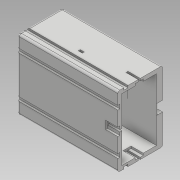
# Autodesk Inventor part: case
Saved by Autodesk Inventor 2018.2 (Build 222227000, 227)
## iProperties
Created: 2019-05-28
Part Number: case
Material: Generico
Document SubType Name: Modeling
Designer: fabio
Density: 1 g/cm^3
Appearance: Default
Author: fabio
Autodesk Inventor part; units mm, degrees
ref_plane "YZ Plane" through (0, 0, 0) normal (1, 0, 0) x (0, 1, 0)
ref_plane "XZ Plane" through (0, 0, 0) normal (0, 1, 0) x (-1, 0, 0)
ref_plane "XY Plane" through (0, 0, 0) normal (0, 0, 1) x (1, 0, 0)
sketch "Schizzo1" plane through (0, 0, 0) normal (0, 1, 0) x (-1, 0, 0)
  line L0 (-20.2, 15.3) -> (20.2, 15.3)
  line L1 (20.2, 15.3) -> (20.2, -15.3)
  line L2 (20.2, -15.3) -> (-20.2, -15.3)
  line L3 (-20.2, -15.3) -> (-20.2, 15.3)
  line L4 (-20.2, 15.3) -> (20.2, -15.3) construction
  line L5 (20.2, 15.3) -> (-20.2, -15.3) construction
  line L6 (20.2, 13.3) -> (-20.2, 13.3)
  line L7 (20.2, 2.3) -> (20.2, 15.3)
  line L8 (20.2, 15.3) -> (15.7, 15.3)
  line L9 (15.7, 15.3) -> (15.7, 2.3)
  line L10 (15.7, 2.3) -> (20.2, 2.3)
  line L11 (20.2, -9.3) -> (20.2, -15.3)
  line L12 (20.2, -15.3) -> (15.7, -15.3)
  line L13 (15.7, -15.3) -> (15.7, -9.3)
  line L14 (15.7, -9.3) -> (20.2, -9.3)
  line L15 (20.2, 15.3) -> (20.2, 12.3)
  line L16 (20.2, 12.3) -> (2.7, 12.3)
  line L17 (2.7, 12.3) -> (2.7, 15.3)
  line L18 (2.7, 15.3) -> (20.2, 15.3)
  point P0 (0, 0)
  dimension "d0" = 40.4
  dimension "d1" = 30.6
  dimension "d2" = 2
  dimension "d3" = 4.5
  dimension "d4" = 13
  dimension "d5" = 4.5
  dimension "d6" = 6
  dimension "d19" = 3
  dimension "d20" = 17.5
  constraints: 38 end point, 8 parallel, 7 perpendicular, 5 point on line, 2 midpoint, 1 horizontal
  measures "d0" distance of L1.end L2.end
  measures "d1" distance of L2.end L0.start
  measures "d2" distance between parallel lines of L6 L0
  measures "d3" distance of L9.end L7.start
  measures "d4" distance of L8.end L9.end
  measures "d5" distance of L13.end L11.start
  measures "d6" distance of L12.end L13.end
  measures "d19" distance of L16.end L17.end
  measures "d20" distance between parallel lines of L17 L7
extrude "Estrusione1" add sketch "Schizzo1" along normal mid plane 4 contours L0 L17 L6 L3 | L0 L9 L6 L17 | L0 L1 L6 L9 | L6 L9 L16 L17 | L6 L1 L16 L9 | L13 L14 L1 L2 | L16 L1 L10 L9
sketch "Schizzo6" plane through (-20.2, 2, 15.3) normal (0, 0, 1) x (1, 0, 0)
  line L0 (0, 0) -> (0, -4) projected
  line L1 (40.4, 0) -> (40.4, -4) projected
  line L2 (0, -4) -> (0, 0) projected
  line L3 (40.4, -3) -> (0, -3)
  line L4 (0, -3) -> (0, -1)
  line L5 (0, -1) -> (40.4, -1)
  line L6 (40.4, -1) -> (40.4, -3)
  line L7 (40.4, -3) -> (0, -1) construction
  line L8 (0, -3) -> (40.4, -1) construction
  point P0 (20.2, -2)
  dimension "d111" = 2
  constraints: 12 end point, 2 midpoint, 2 parallel, 1 horizontal, 1 perpendicular, 1 point on line
  measures "d111" distance between parallel lines of L3 L5
extrude "Estrusione5" cut sketch "Schizzo6" against normal up to surface (30.6 mm away)
sketch "Schizzo7" plane through (0, 2, 0) normal (0, 1, 0) x (1, 0, 0)
  line L0 (-20.2, -15.3) -> (20.2, -15.3) projected
  line L1 (-20.2, -2.3) -> (-20.2, -15.3) projected
  line L2 (-20.2, 15.3) -> (-20.2, 9.3) projected
  line L3 (-15.7, 15.3) -> (-20.2, 15.3) projected
  line L4 (20.2, -15.3) -> (-20.2, -15.3) projected
  line L5 (-20.2, -15.3) -> (20.2, -15.3)
  line L6 (20.2, -15.3) -> (20.2, -17.3)
  line L7 (20.2, -17.3) -> (-20.2, -17.3)
  line L8 (-20.2, -17.3) -> (-20.2, -15.3)
  line L9 (20.2, -13.3) -> (-2.7, -13.3) projected
  line L10 (-20.2, 15.3) -> (-15.7, 15.3) projected
  line L11 (-20.2, 15.3) -> (20.2, 15.3)
  line L12 (20.2, 15.3) -> (20.2, 17.3)
  line L13 (20.2, 17.3) -> (-20.2, 17.3)
  line L14 (-20.2, 17.3) -> (-20.2, 15.3)
  line L15 (-20.2, -17.3) -> (-20.2, 17.3)
  line L16 (-20.2, 17.3) -> (-22.2, 17.3)
  line L17 (-22.2, 17.3) -> (-22.2, -17.3)
  line L18 (-22.2, -17.3) -> (-20.2, -17.3)
  point P0 (0, 0)
  dimension "d25" = 2
  dimension "d26" = 2
  dimension "d27" = 2
  constraints: 24 end point, 7 parallel, 3 perpendicular, 2 collinear
  measures "d25" distance of L0.end L6.end
  measures "d26" distance of L11.end L12.end
  measures "d27" distance of L13.end L16.end
extrude "Estrusione6" add sketch "Schizzo7" against normal up to surface (4 mm away)
sketch "Schizzo10" plane through (-20.2, 2, 2.3) normal (1, 0, 0) x (0, 0, -1)
  line L0 (11.6, -4) -> (11.6, -3) projected
  line L1 (11.6, -4) -> (11.6, -3)
  line L2 (11.6, -3) -> (9.6, -3)
  line L3 (9.6, -3) -> (9.6, -4)
  line L4 (9.6, -4) -> (11.6, -4)
  line L5 (11.6, -3) -> (17.6, -3) projected
  point P0 (2.3, -2)
  dimension "d33" = 2
  dimension "d130" = 1
  constraints: 8 end point, 2 parallel, 2 point on line, 1 perpendicular, 2 other
  measures "d33" distance of L3.end L1.start
  measures "d130" distance of L2.end L3.end
extrude "Estrusione8" cut sketch "Schizzo10" against normal up to surface (2 mm away)
sketch "Schizzo12" plane through (-22.2, 2, 17.3) normal (0, 0, 1) x (1, 0, 0)
  line L0 (42.4, 0) -> (42.4, -4) projected
  line L1 (42.4, 0) -> (42.4, -4) projected
  line L2 (22.4, -3) -> (24.4, -3)
  line L3 (24.4, -3) -> (24.4, -4)
  line L4 (24.4, -4) -> (22.4, -4)
  line L5 (22.4, -4) -> (22.4, -3)
  line L6 (42.4, -3) -> (2, -3) projected
  point P0 (22.2, -2)
  dimension "d42" = 18
  dimension "d43" = 2
  dimension "d44" = 1
  constraints: 8 end point, 2 parallel, 1 horizontal, 1 perpendicular, 1 other
  measures "d42" distance between parallel lines of L0 L3
  measures "d43" distance of L3.end L4.end
  measures "d44" distance of L4.end L2.start
extrude "Estrusione10" cut sketch "Schizzo12" against normal up to surface (4 mm away)
sketch "Schizzo13" plane through (20.2, 1, 13.3) normal (1, 0, 0) x (0, 0, -1)
  line L0 (-4, 1) -> (0, 1) projected
  line L1 (28.6, 1) -> (30.6, 1) projected
  line L2 (-4, 1) -> (-4, -3) projected
  line L3 (-2, 0) -> (-2, -2) projected
  line L4 (-4, 1) -> (-2, 1)
  line L5 (-2, 1) -> (-2, 8.5)
  line L6 (-2, 8.5) -> (-4, 8.5)
  line L7 (-4, 8.5) -> (-4, 1)
  line L8 (-2, -2) -> (-2, 1)
  line L9 (22.6, 1) -> (28.6, 1) projected
  line L10 (28.6, 1) -> (30.6, 1)
  line L11 (30.6, 1) -> (30.6, 8.5)
  line L12 (30.6, 8.5) -> (28.6, 8.5)
  line L13 (28.6, 8.5) -> (28.6, 1)
  line L14 (-4, 8.5) -> (30.6, 8.5)
  line L15 (30.6, 8.5) -> (30.6, 11.5)
  line L16 (30.6, 11.5) -> (-4, 11.5)
  line L17 (-4, 11.5) -> (-4, 8.5)
  point P0 (13.3, -1)
  dimension "d47" = 10.5
  dimension "d48" = 3
  constraints: 26 end point, 6 parallel, 4 perpendicular, 2 collinear, 1 midpoint
  measures "d47" distance from line of L3.end L6
  measures "d48" distance of L11.end L15.end
extrude "Estrusione11" add sketch "Schizzo13" against normal up to surface (42.4 mm away)
sketch "Schizzo15" plane through (20.2, -2, 13.3) normal (1, 0, 0) x (0, 0, -1)
  line L0 (0, 0) -> (-4, 0) projected
  line L1 (-2, 3) -> (-2, 1) projected
  line L2 (28.6, 0) -> (30.6, 0) projected
  line L3 (-4, 0) -> (-2, 0)
  line L4 (-2, 0) -> (-2, -5.5)
  line L5 (-2, -5.5) -> (-4, -5.5)
  line L6 (-4, -5.5) -> (-4, 0)
  line L7 (-2, 1) -> (-2, 0)
  line L8 (28.6, 11.5) -> (28.6, 0) projected
  line L9 (28.6, 0) -> (30.6, 0)
  line L10 (30.6, 0) -> (30.6, -5.5)
  line L11 (30.6, -5.5) -> (28.6, -5.5)
  line L12 (28.6, -5.5) -> (28.6, 0)
  line L13 (-4, -5.5) -> (30.6, -5.5)
  line L14 (30.6, -5.5) -> (30.6, -7.5)
  line L15 (30.6, -7.5) -> (-4, -7.5)
  line L16 (-4, -7.5) -> (-4, -5.5)
  point P0 (13.3, 2)
  dimension "d53" = 8.5
  dimension "d54" = 2
  constraints: 26 end point, 6 parallel, 4 perpendicular, 2 collinear, 1 midpoint
  measures "d53" distance from line of L5 L1.start
  measures "d54" distance of L10.end L14.end
extrude "Estrusione13" add sketch "Schizzo15" against normal up to surface (42.4 mm away)
sketch "Schizzo14" plane through (0, 2, 0) normal (0, 1, 0) x (1, 0, 0)
  line L0 (-22.2, 15.3) -> (-22.2, -15.3) projected
  line L1 (-15.7, 15.3) -> (-22.2, 15.3) projected
  line L2 (-22.2, -15.3) -> (20.2, -15.3) projected
  line L3 (-20.2, -2.3) -> (-20.2, 9.3) projected
  line L4 (-22.2, 15.3) -> (-22.2, -15.3)
  line L5 (-22.2, -15.3) -> (-20.2, -15.3)
  line L6 (-20.2, -15.3) -> (-20.2, 15.3)
  line L7 (-20.2, 15.3) -> (-22.2, 15.3)
  point P0 (0, 0)
  constraints: 8 end point, 3 equal length, 1 collinear, 1 perpendicular
extrude "Estrusione14" add sketch "Schizzo14" along normal up to surface (7.5 mm away)
sketch "Schizzo16" plane through (0, -2, 0) normal (0, -1, 0) x (1, 0, 0)
  line L0 (-22.2, -15.3) -> (-22.2, 15.3) projected
  line L1 (-20.2, 2.3) -> (-20.2, -7.3) projected
  line L2 (-22.2, -15.3) -> (-15.7, -15.3) projected
  line L3 (20.2, 15.3) -> (-22.2, 15.3) projected
  line L4 (-22.2, -15.3) -> (-22.2, 15.3)
  line L5 (-22.2, 15.3) -> (-20.2, 15.3)
  line L6 (-20.2, 15.3) -> (-20.2, -15.3)
  line L7 (-20.2, -15.3) -> (-22.2, -15.3)
  point P0 (0, 0)
  point P1 (-20.2, -9.2)
  constraints: 8 end point, 2 parallel, 1 collinear, 1 perpendicular, 1 vertical
extrude "Estrusione15" add sketch "Schizzo16" along normal up to surface (5.5 mm away)
sketch "Schizzo20" plane through (20.2, 12.5, 17.3) normal (1, 0, 0) x (0, 0, -1)
  line L0 (34.6, 0) -> (0, 0) projected
  line L1 (0, 0) -> (0, -22) projected
  line L2 (0, -22) -> (34.6, -22) projected
  line L3 (32.6, -20) -> (2, -20) projected
  line L4 (2, -20) -> (2, -14.5) projected
  line L5 (2, -10.5) -> (2, -3) projected
  line L6 (2, -3) -> (32.6, -3) projected
  line L7 (32.6, -3) -> (32.6, -20) projected
  line L8 (34.6, -22) -> (34.6, 0) projected
  line L9 (2, -10.5) -> (2, -14.5)
  point P0 (17.3, -12.5)
  constraints: 2 end point
extrude "Estrusione17" add sketch "Schizzo20" along normal blind 7
sketch "Schizzo26" plane through (27.2, 12.5, 17.3) normal (1, 0, 0) x (0, 0, -1)
  line L0 (2, -3) -> (32.6, -3) projected
  line L1 (2, -20) -> (2, -3) projected
  line L2 (32.6, -20) -> (2, -20) projected
  line L3 (32.6, -3) -> (32.6, -20) projected
  line L4 (2, -3) -> (32.6, -3) projected
  line L5 (17.3, -3) -> (17.3, -20)
  line L6 (32.6, -20) -> (2, -20) projected
  line L7 (2, -11.5) -> (17.3, -11.5)
  line L8 (17.3, -11.5) -> (32.6, -11.5)
  line L9 (17.8, -3) -> (16.8, -3)
  line L10 (16.8, -3) -> (16.8, -2)
  line L11 (16.8, -2) -> (15.3, -2)
  line L12 (15.3, -2) -> (15.3, -1)
  line L13 (15.3, -1) -> (19.3, -1)
  line L14 (19.3, -1) -> (19.3, -2)
  line L15 (19.3, -2) -> (17.8, -2)
  line L16 (17.8, -2) -> (17.8, -3)
  line L17 (17.8, -20) -> (16.8, -20)
  line L18 (16.8, -20) -> (16.8, -21)
  line L19 (16.8, -21) -> (15.3, -21)
  line L20 (15.3, -21) -> (15.3, -22)
  line L21 (15.3, -22) -> (19.3, -22)
  line L22 (19.3, -22) -> (19.3, -21)
  line L23 (19.3, -21) -> (17.8, -21)
  line L24 (17.8, -21) -> (17.8, -20)
  line L25 (32.6, -13.5) -> (32.6, -9.5)
  line L26 (32.6, -9.5) -> (33.6, -9.5)
  line L27 (33.6, -9.5) -> (33.6, -11)
  line L28 (33.6, -11) -> (34.6, -11)
  line L29 (34.6, -11) -> (34.6, -12)
  line L30 (34.6, -12) -> (33.6, -12)
  line L31 (33.6, -12) -> (33.6, -13.5)
  line L32 (33.6, -13.5) -> (32.6, -13.5)
  line L33 (2, -13.5) -> (2, -9.5)
  line L34 (2, -9.5) -> (1, -9.5)
  line L35 (1, -9.5) -> (1, -11)
  line L36 (1, -11) -> (0, -11)
  line L37 (0, -11) -> (0, -12)
  line L38 (0, -12) -> (1, -12)
  line L39 (1, -12) -> (1, -13.5)
  line L40 (1, -13.5) -> (2, -13.5)
  point P0 (17.3, -12.5)
  dimension "d82" = 1
  dimension "d83" = 1
  dimension "d84" = 1
  dimension "d85" = 4
  dimension "d86" = 1.5
  dimension "d87" = 4
  dimension "d88" = 1
  dimension "d89" = 1
  dimension "d91" = 1
  dimension "d94" = 1.5
  constraints: 70 end point, 16 symmetric about line, 12 perpendicular, 9 midpoint, 8 point on line, 1 horizontal, 1 vertical
  measures "d82" distance of L15.end L9.start
  measures "d83" distance of L13.end L14.end
  measures "d84" distance of L9.start L9.end
  measures "d85" distance of L12.end L13.end
  measures "d86" distance of L10.end L11.end
  measures "d87" distance of L25.start L25.end
  measures "d88" distance of L31.end L25.start
  measures "d89" distance of L29.end L30.end
  measures "d91" distance of L28.end L29.end
  measures "d94" distance of L26.end L27.end
extrude "Estrusione29" cut sketch "Schizzo26" against normal blind 6 contours L1 L40 L39 L38 L37 L36 L35 L34 | L2 L24 L23 L22 L21 L20 L19 L18 | L3 L26 L27 L28 L29 L30 L31 L32
sketch "Schizzo35" plane through (27.2, 12.5, 17.3) normal (1, 0, 0) x (0, 0, -1)
  line L0 (34.6, 0) -> (0, 0) projected
  line L1 (14.8, 0) -> (19.8, 0)
  line L2 (19.8, 0) -> (19.8, -2)
  line L3 (19.8, -2) -> (14.8, -2)
  line L4 (14.8, -2) -> (14.8, 0)
  point P0 (17.3, -12.5)
  point P1 (17.3, 0)
  dimension "d119" = 5
  dimension "d120" = 2
  constraints: 8 end point, 2 midpoint, 2 parallel, 1 horizontal, 1 perpendicular
  measures "d119" distance of L2.end L3.end
  measures "d120" distance of L1.end L2.end
extrude "Estrusione30" cut sketch "Schizzo35" against normal blind 15
sketch "Schizzo36" plane through (27.2, 10.5, 2.5) normal (0, 0, -1) x (-1, 0, 0)
  line L0 (0, 0) -> (15, 0) projected
  line L1 (14.1, 0) -> (14.1, -0.9)
  arc A0 (14.1, -0.9) -> (15, 0) centre (14.1, 0) ccw
  point P0 (27.2, -10.5)
  dimension "d123" = 0.9
  constraints: 2 end point, 2 point on circle, 1 centre point, 1 coincident, 1 point on line, 1 vertical
  measures "d123" distance of L1.start L1.end
extrude "Estrusione31" cut sketch "Schizzo36" along normal up to surface (5 mm away)
sketch "Schizzo28" plane through (27.2, 12.5, 17.3) normal (1, 0, 0) x (0, 0, -1)
  line L0 (0, -22) -> (34.6, -22) projected
  line L1 (0, -22) -> (34.6, -22) projected
  line L2 (0, 0) -> (0, -22) projected
  line L3 (6, -22) -> (8, -22)
  line L4 (8, -22) -> (8, -21)
  line L5 (8, -21) -> (6, -21)
  line L6 (6, -21) -> (6, -22)
  line L7 (16.7, -19) -> (17.7, -19) projected
  line L8 (17.3, -12.5) -> (17.3, -20)
  line L9 (32.6, -20) -> (2, -20) projected
  line L10 (0, 0) -> (0, -22) projected
  line L11 (0, -19) -> (0, -17)
  line L12 (0, -17) -> (1, -17)
  line L13 (1, -17) -> (1, -19)
  line L14 (1, -19) -> (0, -19)
  line L15 (28.6, -22) -> (26.6, -22)
  line L16 (26.6, -22) -> (26.6, -21)
  line L17 (26.6, -21) -> (28.6, -21)
  line L18 (28.6, -21) -> (28.6, -22)
  line L19 (34.6, -17) -> (33.6, -17)
  line L20 (33.6, -17) -> (33.6, -19)
  line L21 (33.6, -19) -> (34.6, -19)
  line L22 (34.6, -17) -> (34.6, -19)
  line L23 (34.6, -22) -> (34.6, 0) projected
  point P0 (15.2, -21)
  point P1 (19.2, -21)
  point P2 (0, -11)
  point P3 (34.4, -11)
  point P4 (2, -20)
  point P5 (34.6, 0)
  dimension "d95" = 2
  dimension "d96" = 1
  dimension "d97" = 1
  dimension "d98" = 2
  dimension "d99" = 3
  dimension "d129" = 6
  constraints: 34 end point, 8 symmetric about line, 4 parallel, 2 perpendicular, 2 point on line, 1 vertical, 7 other
  measures "d95" distance between parallel lines of L4 L6
  measures "d96" distance of L5.end L3.start
  measures "d97" distance of L13.end L11.start
  measures "d98" distance between parallel lines of L14 L12
  measures "d129" distance between parallel lines of L2 L6
extrude "Estrusione23" cut sketch "Schizzo28" against normal up to surface (49.4 mm away)
sketch "Schizzo37" plane through (-22.2, 12.5, 17.3) normal (0, 1, 0) x (1, 0, 0)
  line L0 (34.4, 14.8) -> (34.4, 19.8) projected
  line L1 (34.4, 9.8) -> (34.4, 24.8)
  arc A0 (34.4, 24.8) -> (34.4, 9.8) centre (34.4, 17.3) ccw
  point P0 (22.2, 17.3)
  dimension "d126" = 15
  constraints: 2 end point, 2 midpoint, 2 point on circle, 1 centre point, 1 coincident, 1 collinear, 1 vertical
  measures "d126" distance of L1.start L1.end
extrude "Estrusione32" cut sketch "Schizzo37" against normal blind 2.5
sketch "Schizzo39" plane through (12.2, 12.5, -7.5) normal (-1, 0, 0) x (0, 0, 1)
  line L0 (5, -2) -> (10, -2) projected
  line L1 (0, -2.5) -> (15, -2.5) projected
  line L2 (5, -2) -> (5, -2.5)
  line L3 (10, -2) -> (10, -2.9) projected
  line L4 (10, -2) -> (10, -2.5)
  point P0 (7.5, -12.5)
  point P1 (10, -3)
  constraints: 4 end point, 3 point on line, 1 perpendicular
extrude "Estrusione34" cut sketch "Schizzo39" against normal up to surface
fillet "Raccordo2" radius 0.5 14 edges at (20.2, 1, 14.3) (8.75, 1, 13.3) (-2.7, 1, 12.8) (-9.2, 1, 12.3) (-15.7, 1, 7.3) (20.2, -1, 14.3) (11.2, -1, 13.3) (0.2, -1, 14.3) (-1.25, -1, 13.3) (-2.7, -1, 12.8) (-9.2, -1, 12.3) (-15.7, -1, 7.3) (-15.7, -1, -12.3) (-15.7, 1, -12.3)
fillet "Raccordo3" radius 1 1 edges at (27.2, 10.5, 0)
fillet "Raccordo4" radius 1 12 edges at (-22.2, 4, 17.3) (-22.2, 4, -17.3) (-22.2, -9.5, -14.3) (2.5, -9.5, -17.3) (2.5, -9.5, 17.3) (2.5, 12.5, 17.3) (2.5, 12.5, -17.3) (-22.2, 12.5, 0) (-22.2, -9.5, 0) (-22.2, -9.5, 14.3) (-22.2, -8, -17.3) (-22.2, -8, 17.3)
fillet "Raccordo5" radius 2 3 edges at (4.7, 12.5, 0) (12.2, 12.5, 5) (12.2, 12.5, -5)
equation "\"d5\" = d3"
equation "\"d26\" = d25"
equation "\"d27\" = d25"
equation "\"d83\" = d82"
equation "\"d89\" = d88"
equation "\"d98\" = d95"
